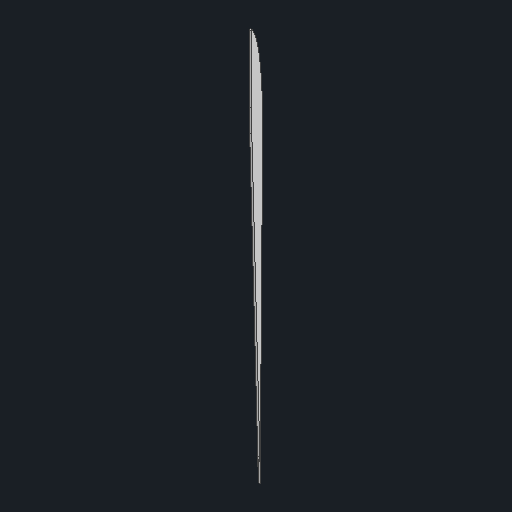
# Autodesk Inventor part: standoff
Saved by Autodesk Inventor 2023 (Build 270158030, 158C)
## iProperties
Created: 2022-03-24
Part Number: standoff
Material: Generic
Document SubType Name: Modeling
Designer: kardo
Density: 1 g/cm^3
Appearance: Default
Author: kardo
Autodesk Inventor part; units mm, degrees
ref_plane "YZ Plane" through (0, 0, 0) normal (1, 0, 0) x (0, 1, 0)
ref_plane "XZ Plane" through (0, 0, 0) normal (0, 1, 0) x (-1, 0, 0)
ref_plane "XY Plane" through (0, 0, 0) normal (0, 0, 1) x (1, 0, 0)
derived "parameters_frame.ipt"
derived "surface_body.ipt"
sketch "sk_rail_bottom_standoff" plane through (34.32, 0, 0) normal (1, 0, 0) x (0, 1, 0)
  line L0 (-363, 18.496) -> (-275.8801, 20.463)
  arc A0 (-275.8801, 20.463) -> (-254.1001, 21.0191) centre (-359.1231, 3707.4463) ccw
  line L1 (30.81, 28.832) -> (94.8, 28.832)
  arc A1 (30.81, 28.832) -> (9.48, 28.5282) centre (30.81, -720.1791) ccw
  line L2 (-254.1001, 21.0191) -> (9.48, 28.5282)
  line L3 (-483, 0) -> (357, 0) construction
  line L4 (9.48, 28.5282) -> (9.48, 0) construction
  line L5 (-254.1001, 21.0191) -> (-254.1001, 0) construction
  point P0 (0, 0)
  point P1 (-254.1001, 20.9547)
  point P2 (9.48, 28.832)
sketch "sk_rail_standoff_standoff" plane through (34.32, 0, 0) normal (1, 0, 0) x (0, 1, 0)
  line L0 (0, 18.496) -> (77.736, 17.8469) construction
  line L1 (77.736, 17.8469) -> (94.8, 28.832) construction
  line L2 (0, 18.496) -> (-254.1001, 20.6178)
  line L3 (-275.8801, 20.463) -> (-363, 18.496)
  arc A0 (-254.1001, 20.6178) -> (-275.8801, 20.463) centre (-259.9816, -683.7109) ccw
  line L4 (-483, 0) -> (357, 0) construction
  line L5 (-254.1001, 20.6178) -> (-254.1001, 0) construction
  spline S0 degree 2 poles (0, 18.496) (77.736, 17.8469) (94.8, 28.832) knots 1 1 1 2 2 2
  point P0 (0, 0)
  point P1 (-254.1001, 20.9547)
ref_plane "plane_standoff_right" through (34.32, 0, 0) normal (1, 0, 0) x (0, 1, 0)
sketch "sk_base" plane through (34.32, 0, 0) normal (1, 0, 0) x (0, 1, 0)
  arc A0 (-254.1001, 20.6178) -> (-275.8801, 20.463) centre (-259.9816, -683.7109) ccw construction
  arc A1 (-275.8801, 20.463) -> (-254.1001, 21.0191) centre (-359.1231, 3707.4463) ccw construction
  line L0 (-254.1001, 21.0191) -> (9.48, 28.5282) construction
  line L1 (0, 18.496) -> (-254.1001, 20.6178) construction
  spline S0 degree 2 poles (0, 18.496) (77.736, 17.8469) (94.8, 28.832) knots 1 1 1 2 2 2 construction
  line L2 (30.81, 28.832) -> (94.8, 28.832) construction
  arc A2 (30.81, 28.832) -> (9.48, 28.5282) centre (30.81, -720.1791) ccw construction
  line L3 (0.01, 19.696) -> (-254.0901, 21.8178)
  arc A3 (-254.0901, 21.8178) -> (-275.8801, 21.6633) centre (-259.9816, -683.7109) ccw
  arc A4 (-275.8801, 21.6633) -> (-254.1343, 22.2186) centre (-359.1231, 3707.4463) ccw
  line L4 (-254.1343, 22.2186) -> (9.4458, 29.7277)
  arc A5 (30.81, 30.032) -> (9.4458, 29.7277) centre (30.81, -720.1791) ccw
  line L5 (30.81, 30.032) -> (92.8, 30.032)
  line L6 (-275.8801, 20.463) -> (-275.8801, 21.6633) construction
  line L7 (92.8, 29.0452) -> (92.8, 30.032)
  spline S1 degree 5 poles (92.8, 29.0452) (91.3624, 28.2663) (89.8576, 27.611) (88.3274, 27.0332) (84.0631, 25.6206) (79.6899, 24.5827) (76.8919, 24.0154) (70.3392, 22.8692) (63.737, 22.0476) (59.9602, 21.6525) (51.4388, 20.8998) (42.8984, 20.4036) (38.1461, 20.1879) (27.6694, 19.8244) (17.1873, 19.6713) (11.4614, 19.6381) (5.7356, 19.6482) (0.01, 19.696) knots 0 0 0 0 0 0 0.087125 0.087125 0.087125 0.239175 0.239175 0.239175 0.441476 0.441476 0.441476 0.694926 0.694926 0.694926 1 1 1 1 1 1
  point P0 (0, 0)
  dimension "d5" = 1.2
  dimension "d4" = 1.2
  dimension "d6" = 2
  constraints: 10 end point, 6 point on circle, 3 centre point, 2 vertical, 1 parallel, 7 other
  measures "d4" distance between parallel lines of L0 L4
  measures "d6" distance from line of L7 point (94.8, 28.832)
extrude "thicken" add sketch "sk_base" against normal blind 2
equation "\"d4\" = shell_thickness"
equation "\"d6\" = bulkhead_thickness"
equation "\"d2\" = bulkhead_thickness"
equation "\"shell_thickness\" = 1.2"
equation "\"bulkhead_thickness\" = 2"
body "Solid1"
